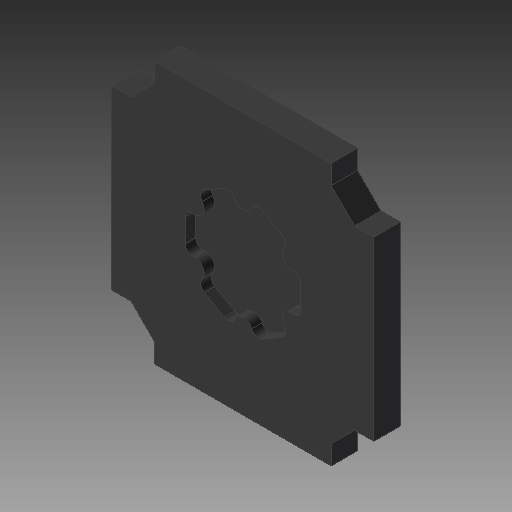
# Autodesk Inventor part: 20_Cube_insert_Sample_holder
Saved by Autodesk Inventor 2019 (Build 230136000, 136)
## iProperties
Created: 2019-08-07
Part Number: 20_Cube_insert_Sample_holder
Material: Generic
Document SubType Name: Modeling
Designer: marsikovabarbora
Density: 1 g/cm^3
Appearance: Default
Author: marsikovabarbora
Autodesk Inventor part; units mm, degrees
ref_plane "YZ Plane" through (0, 0, 0) normal (1, 0, 0) x (0, 1, 0)
ref_plane "XZ Plane" through (0, 0, 0) normal (0, 1, 0) x (-1, 0, 0)
ref_plane "XY Plane" through (0, 0, 0) normal (0, 0, 1) x (1, 0, 0)
sketch "Sketch1" plane through (0, 0, 0) normal (0, 0, 1) x (1, 0, 0)
  line L0 (-34.86, 0) -> (34.86, 0) construction
  line L1 (0, -34.86) -> (0, 34.86) construction
  line L2 (0, 0) -> (11.1575, 11.1575) construction
  line L3 (0, 0) -> (15.7791, 0) construction
  line L4 (0, 24.9) -> (16.8009, 24.9)
  line L5 (16.8009, 24.9) -> (16.8009, 21.2415)
  line L6 (16.8009, 21.2415) -> (19.0212, 19.0212)
  line L7 (24.9, 0) -> (24.9, 16.8009)
  line L8 (24.9, 16.8009) -> (21.2415, 16.8009)
  line L9 (21.2415, 16.8009) -> (19.0212, 19.0212)
  line L10 (0, -24.9) -> (16.8009, -24.9)
  line L11 (16.8009, -24.9) -> (16.8009, -21.2415)
  line L12 (16.8009, -21.2415) -> (19.0212, -19.0212)
  line L13 (24.9, 0) -> (24.9, -16.8009)
  line L14 (24.9, -16.8009) -> (21.2415, -16.8009)
  line L15 (21.2415, -16.8009) -> (19.0212, -19.0212)
  line L16 (0, 24.9) -> (-16.8009, 24.9)
  line L17 (-16.8009, 24.9) -> (-16.8009, 21.2415)
  line L18 (-16.8009, 21.2415) -> (-19.0212, 19.0212)
  line L19 (-24.9, 16.8009) -> (-21.2415, 16.8009)
  line L20 (-21.2415, 16.8009) -> (-19.0212, 19.0212)
  line L21 (0, -24.9) -> (-16.8009, -24.9)
  line L22 (-16.8009, -24.9) -> (-16.8009, -21.2415)
  line L23 (-16.8009, -21.2415) -> (-19.0212, -19.0212)
  line L24 (-21.2415, -16.8009) -> (-19.0212, -19.0212)
  line L25 (-24.9, -16.8009) -> (-21.2415, -16.8009)
  line L26 (-24.9, 0) -> (-24.9, -16.8009)
  line L27 (-24.9, 0) -> (-24.9, 16.8009)
  circle A0 centre (0, 0) radius 12.5
  dimension "d0" = 45
  dimension "d2" = 24.9
  dimension "d3" = 3.14
  dimension "d4" = 26.9
  dimension "d5" = 25
  constraints: 52 end point, 20 symmetric about line, 2 horizontal, 2 perpendicular, 2 point on line, 1 centre point, 1 coincident, 1 equal length
  measures "d0" angle of L3 L2
  measures "d2" distance between parallel lines of L0 L4
  measures "d3" distance of L5.end L6.end
  measures "d4" distance from line of L2.start L6
  measures "d5" diameter of A0
extrude "Extrusion1" add sketch "Sketch1" along normal blind 5
sketch "Sketch3" plane through (0, 0, 0) normal (0, 0, -1) x (-1, 0, 0)
  circle A0 centre (0, 0) radius 12.5 projected
extrude "Extrusion3" add sketch "Sketch3" against normal blind 3
sketch "Sketch4" plane through (0, 0, 3) normal (0, 0, 1) x (1, 0, 0)
  circle A0 centre (0, 0) radius 12.5 projected
  arc A1 (-2.4955, 9.5466) -> (0.05, 7.811) centre (0.05, 10.5454) ccw projected
  arc A2 (-2.4955, 9.5466) -> (-3.0679, 9.7469) centre (-2.8679, 9.4005) ccw projected
  line L0 (-3.0679, 9.7469) -> (-6.8321, 7.5736) projected
  arc A3 (-6.8321, 7.5736) -> (-6.9449, 6.9778) centre (-6.6321, 7.2272) ccw projected
  arc A4 (-6.7145, 3.9055) -> (-6.9449, 6.9778) centre (-9.0826, 5.2727) ccw projected
  arc A5 (2.5955, -9.5466) -> (0.05, -7.811) centre (0.05, -10.5454) ccw projected
  arc A6 (2.5955, -9.5466) -> (3.1679, -9.7469) centre (2.9679, -9.4005) ccw projected
  line L1 (3.1679, -9.7469) -> (6.9321, -7.5736) projected
  arc A7 (6.9321, -7.5736) -> (7.0449, -6.9778) centre (6.7321, -7.2272) ccw projected
  arc A8 (6.8145, -3.9055) -> (7.0449, -6.9778) centre (9.1826, -5.2727) ccw projected
  line L2 (5.3229, -1.93) -> (5.3229, -1.58) projected
  line L3 (5.3229, -1.58) -> (5.4719, -1.58) projected
  line L4 (6.0377, -2.56) -> (5.9268, -2.56) projected
  line L5 (5.9268, -2.56) -> (5.9268, -2.3679) projected
  line L6 (5.674, -1.93) -> (5.3229, -1.93) projected
  circle A9 centre (0.05, 0) radius 3.3699 projected
  line L7 (1.2704, -6.4878) -> (4.6724, -4.4373) projected
  line L8 (4.6724, -4.4373) -> (5.9738, -6.5964) projected
  line L9 (5.9738, -6.5964) -> (2.5718, -8.647) projected
  line L10 (2.5718, -8.647) -> (1.2704, -6.4878) projected
  line L11 (-2.4718, 8.647) -> (-1.1704, 6.4878) projected
  line L12 (-1.1704, 6.4878) -> (-4.5724, 4.4373) projected
  line L13 (-4.5724, 4.4373) -> (-5.8738, 6.5964) projected
  line L14 (-5.8738, 6.5964) -> (-2.4718, 8.647) projected
  arc A10 (-3.5679, -10.6129) -> (-1.5646, -9.9119) centre (-2.8679, -9.4005) ccw
  line L15 (-3.5679, -10.6129) -> (-7.3321, -8.4396)
  arc A11 (-7.7266, -6.3542) -> (-7.3321, -8.4396) centre (-6.6321, -7.2272) ccw
  arc A12 (-7.7266, -6.3542) -> (-9.3412, -3.5577) centre (-9.0826, -5.2727) ccw
  arc A13 (-10.95, -2.1733) -> (-9.3412, -3.5577) centre (-9.55, -2.1733) ccw
  line L16 (-10.95, -2.1733) -> (-10.95, 2.1733)
  arc A14 (-9.3412, 3.5577) -> (-10.95, 2.1733) centre (-9.55, 2.1733) ccw
  arc A15 (-9.3412, 3.5577) -> (-7.7266, 6.3542) centre (-9.0826, 5.2727) ccw
  arc A16 (-7.3321, 8.4396) -> (-7.7266, 6.3542) centre (-6.6321, 7.2272) ccw
  line L17 (-7.3321, 8.4396) -> (-3.5679, 10.6129)
  arc A17 (-1.5646, 9.9119) -> (-3.5679, 10.6129) centre (-2.8679, 9.4005) ccw
  arc A18 (-1.5646, 9.9119) -> (1.6646, 9.9119) centre (0.05, 10.5454) ccw
  arc A19 (3.6679, 10.6129) -> (1.6646, 9.9119) centre (2.9679, 9.4005) ccw
  line L18 (3.6679, 10.6129) -> (7.4321, 8.4396)
  arc A20 (7.8266, 6.3542) -> (7.4321, 8.4396) centre (6.7321, 7.2272) ccw
  arc A21 (7.8266, 6.3542) -> (9.4412, 3.5577) centre (9.1826, 5.2727) ccw
  arc A22 (11.05, 2.1733) -> (9.4412, 3.5577) centre (9.65, 2.1733) ccw
  line L19 (11.05, 2.1733) -> (11.05, -2.1733)
  arc A23 (9.4412, -3.5577) -> (11.05, -2.1733) centre (9.65, -2.1733) ccw
  arc A24 (9.4412, -3.5577) -> (7.8266, -6.3542) centre (9.1826, -5.2727) ccw
  arc A25 (7.4321, -8.4396) -> (7.8266, -6.3542) centre (6.7321, -7.2272) ccw
  line L20 (7.4321, -8.4396) -> (3.6679, -10.6129)
  arc A26 (1.6646, -9.9119) -> (3.6679, -10.6129) centre (2.9679, -9.4005) ccw
  arc A27 (1.6646, -9.9119) -> (-1.5646, -9.9119) centre (0.05, -10.5454) ccw
  line L21 (-6.7145, 3.9055) -> (0.05, -7.811) projected
  line L22 (6.8145, -3.9055) -> (6.0377, -2.56) projected
  line L23 (5.9268, -2.3679) -> (5.674, -1.93) projected
  line L24 (5.4719, -1.58) -> (0.05, 7.811) projected
  dimension "d15" = 1
  constraints: 36 point on circle, 18 centre point, 12 end point, 8 other
  measures "d15" radial gap between concentric circles of A5 A27
extrude "Extrusion4" add sketch "Sketch4" along normal up to surface (2 mm away) contours A0
body "Solid1"
